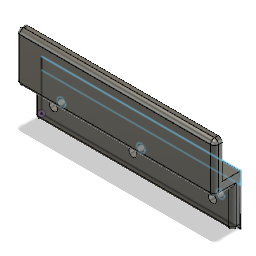
Bottom Bracket (Autodesk Fusion 360 design; units mm, degrees)
Autodesk Fusion 360 part; units mm, degrees
sketch "Sketch1" plane through (0, 0, 0) normal (0, 0, 1) x (1, 0, 0)
  line L0 (0, 0) -> (100, 0)
  line L1 (100, 0) -> (100, 25)
  line L2 (100, 25) -> (0, 25)
  line L3 (0, 25) -> (0, 0)
  line L4 (0, 25) -> (100, 25)
  line L5 (100, 25) -> (100, 19)
  line L6 (100, 19) -> (0, 19)
  line L7 (0, 19) -> (0, 25)
  circle A0 centre (50, 10) radius 2
  circle A1 centre (10, 10) radius 2
  circle A2 centre (90, 10) radius 2
  dimension "d1" = 100
  dimension "d2" = 6
  dimension "d12" = 4
  dimension "d13" = 4
  dimension "d14" = 4
  constraint horizontal L0
  constraint vertical L1
  constraint horizontal L2
  constraint vertical L3
  constraint coincident L0.start L3.end
  constraint horizontal L4
  constraint vertical L5
  constraint horizontal L6
  constraint vertical L7
  measures "d1" distance of L0.start L0.end
  measures "d2" distance of L2.end L6.end L0.start
  measures "d12" diameter of A0
  measures "d13" diameter of A1
  measures "d14" diameter of A2
extrude "Extrude1" add sketch "Sketch1" along normal blind 4 contours L0 L1 L3 L6
extrude "Extrude2" add sketch "Sketch1" along normal blind 9 contours L1 L2 L3 L4 L5 L6 L7
sketch "Sketch2" plane through (0, 0, 9) normal (0, 0, 1) x (1, 0, 0)
  line L0 (0, 19) -> (100, 19)
  line L1 (100, 19) -> (100, 25)
  line L2 (100, 25) -> (0, 25)
  line L3 (0, 25) -> (0, 19)
  line L4 (0, 19) -> (100, 19)
  line L5 (100, 19) -> (100, 44)
  line L6 (100, 44) -> (0, 44)
  line L7 (0, 44) -> (0, 19)
  dimension "d7" = 25
  dimension "d8" = 100
  constraint horizontal L4
  constraint vertical L5
  constraint horizontal L6
  constraint vertical L7
  constraint coincident L0.start L3.end
  measures "d7" distance of L0.start L6.end
  measures "d8" distance of L0.start L0.end
extrude "Extrude3" add sketch "Sketch2" along normal blind 4
fillet "Fillet1" radius 2 13 edges at (50, 44, 13) (0, 31.5, 13) (100, 44, 11) (100, 31.5, 13) (50, 19, 13) (100, 19, 8.5) (100, 9.5, 4) (50, 0, 4) (0, 9.5, 4) (100, 0, 2) (0, 0, 2) (0, 19, 8.5) (0, 44, 11)
